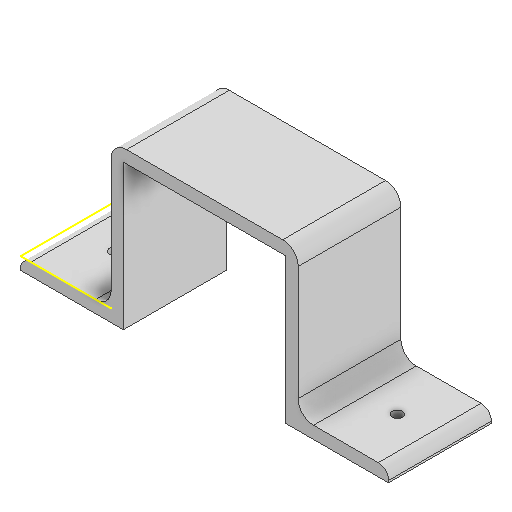
# Autodesk Inventor part: Batterijbevestiging
Saved by Autodesk Inventor 2026.1 (Build 301233020, 233B)
## iProperties
Created: 2026-03-05
Part Number: Batterijbevestiging
Material: Generic
Document SubType Name: Modeling
Designer: senne
Density: 1 g/cm^3
Appearance: Default
Author: senne
Autodesk Inventor part; units mm, degrees
ref_plane "YZ Plane" through (0, 0, 0) normal (1, 0, 0) x (0, 1, 0)
ref_plane "XZ Plane" through (0, 0, 0) normal (0, 1, 0) x (-1, 0, 0)
ref_plane "XY Plane" through (0, 0, 0) normal (0, 0, 1) x (1, 0, 0)
sketch "Sketch1" plane through (0, 0, 0) normal (0, 0, 1) x (1, 0, 0)
  line L0 (-8.9, 0) -> (9.3, 0)
  line L1 (9.3, 0) -> (9.3, -14.13)
  line L2 (-8.9, -14.13) -> (-8.9, 0)
  line L3 (-7.7, -1.2) -> (8.1, -1.2)
  line L4 (8.1, -1.2) -> (8.1, -15.33)
  line L5 (-7.7, -15.33) -> (-7.7, -1.2)
  line L6 (-8.9, -14.13) -> (-17.7, -14.13)
  line L7 (-17.7, -14.13) -> (-17.7, -15.33)
  line L8 (-17.7, -15.33) -> (-7.7, -15.33)
  line L9 (9.3, -14.13) -> (18.1, -14.13)
  line L10 (18.1, -14.13) -> (18.1, -15.33)
  line L11 (18.1, -15.33) -> (8.1, -15.33)
  point P0 (0, 0)
  dimension "d0" = 1.2
  dimension "d1" = 1.2
  dimension "d2" = 1.2
  dimension "d3" = 15.8
  dimension "d4" = 14.13
  dimension "d5" = 10
  dimension "d6" = 10
  dimension "d7" = 1.2
  dimension "d8" = 1.2
  constraints: 24 end point, 5 perpendicular, 4 horizontal, 4 parallel, 1 point on line
  measures "d0" distance between parallel lines of L0 L3
  measures "d1" distance between parallel lines of L1 L4
  measures "d2" distance between parallel lines of L2 L5
  measures "d3" distance of L3.start L3.end
  measures "d4" distance of L3.end L4.end
  measures "d5" distance of L10.end L4.end
  measures "d6" distance of L7.end L5.start
  measures "d7" distance of L9.end L10.end
  measures "d8" distance of L6.end L7.end
extrude "Extrusion1" add sketch "Sketch1" along normal blind 10
sketch "Sketch2" plane through (-17.7, -14.13, 0) normal (0, 1, 0) x (1, 0, 0)
  line L0 (8.8, 0) -> (0, 0) projected
  line L1 (0, 0) -> (0, -10) projected
  line L2 (8.8, -10) -> (0, -10) projected
  line L3 (8.8, 0) -> (8.8, -10) projected
  point P0 (17.7, 0)
fillet "Fillet1" radius 1 2 edges at (18.1, -14.13, 5) (-17.7, -14.13, 5)
fillet "Fillet2" radius 1.5 4 edges at (-8.9, 0, 5) (9.3, 0, 5) (9.3, -14.13, 5) (-8.9, -14.13, 5)
sketch "Sketch3" plane through (-16.7, -14.13, 10) normal (0, 1, 0) x (1, 0, 0)
  circle A0 centre (3.15, 5) radius 0.5
  line L0 (33.8, 0) -> (27.5, 0) projected
  line L1 (27.5, 0) -> (27.5, 10) projected
  line L2 (33.8, 10) -> (27.5, 10) projected
  line L3 (33.8, 10) -> (33.8, 0) projected
  line L4 (27.5, 0) -> (27.5, 10) projected
  line L5 (33.8, 0) -> (27.5, 0) projected
  line L6 (33.8, 10) -> (33.8, 0) projected
  line L7 (33.8, 10) -> (27.5, 10) projected
  line L8 (34.8, 0) -> (33.8, 0) projected
  line L9 (33.8, 10) -> (34.8, 10) projected
  line L10 (34.8, 0) -> (34.8, 10) projected
  line L11 (33.8, 0) -> (34.8, 0) projected
  line L12 (34.8, 0) -> (34.8, 10) projected
  line L13 (34.8, 10) -> (33.8, 10) projected
  line L14 (33.8, 10) -> (33.8, 0) projected
  line L15 (34.8, 10) -> (34.8, 0) projected
  line L16 (34.8, 0) -> (34.8, 10) projected
  line L17 (34.8, 10) -> (34.8, 0) projected
  circle A1 centre (30.65, 5) radius 0.5
  point P0 (16.7, 10)
  dimension "d16" = 1
  dimension "d17" = 1
  constraints: 2 centre point
  measures "d16" diameter of A1
  measures "d17" diameter of A0
extrude "Extrusion2" cut sketch "Sketch3" against normal through all contours A0 | A1
body "Solid1"
